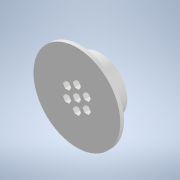
# Autodesk Inventor part: tire vtulka
Saved by Autodesk Inventor 2022 (Build 260153000, 153)
## iProperties
Created: 2023-02-08
Part Number: tire vtulka
Material: Типовые
Document SubType Name: Modeling
Designer: akapu
Density: 1 g/cm^3
Appearance: По умолчанию
Author: akapu
Autodesk Inventor part; units mm, degrees
ref_plane "YZ Plane" through (0, 0, 0) normal (1, 0, 0) x (0, 1, 0)
ref_plane "XZ Plane" through (0, 0, 0) normal (0, 1, 0) x (-1, 0, 0)
ref_plane "XY Plane" through (0, 0, 0) normal (0, 0, 1) x (1, 0, 0)
sketch "Эскиз1" plane through (0, 0, 0) normal (1, 0, 0) x (0, 1, 0)
  line L0 (-3.98, -3) -> (-3.38, 0)
  line L1 (-3.98, -3) -> (-56.02, -3) projected
  line L2 (-4.48, -22.93) -> (-4.48, -3)
  line L3 (-55.52, -22.93) -> (-55.52, -3)
  line L4 (-3.98, -3) -> (-56.02, -3) projected
  line L5 (-56.02, -3) -> (-56.62, 0)
  line L6 (-60, 0) -> (0, 0) projected
  line L7 (-60, 0) -> (-60, -22.93)
  line L8 (0, 0) -> (0, -22.93)
  line L9 (-60, -22.93) -> (0, -22.93) projected
  line L10 (-3.98, -3) -> (-3.98, -3)
  line L11 (-3.98, -3) -> (-3.38, 0)
  line L12 (-56.02, -3) -> (-56.02, -3)
  line L13 (-56.02, -3) -> (-56.62, 0)
  line L14 (-3.38, 0) -> (4.62, 0)
  line L15 (-56.62, 0) -> (-64.62, 0)
  line L16 (-64.62, 0) -> (-64.62, 3)
  line L17 (-64.62, 3) -> (4.62, 3)
  line L18 (4.62, 3) -> (4.62, 0)
  line L19 (-30, -3) -> (-51.25, -3)
  line L20 (-51.25, -3) -> (-8.75, -3)
  line L21 (-8.75, -3) -> (-8.75, -22.93)
  line L22 (-51.25, -3) -> (-51.25, -22.93)
  line L23 (-8.4375, -4) -> (-8.4375, -3)
  line L24 (-8.125, -4) -> (-8.75, -4)
  spline S0 degree 2 poles (-7.5, -3) (-8.8703, -3.1757) (-8.75, -5) knots 0 0 0 1 1 1
  line L25 (-7.5, -3) -> (-8.75, -5)
  line L26 (-7.5, -3) -> (-8.75, -3)
  line L27 (-8.125, -21.93) -> (-8.75, -21.93)
  line L28 (-7.5, -22.93) -> (-8.75, -20.93)
  line L29 (-7.5, -22.93) -> (-8.75, -22.93)
  spline S1 degree 2 poles (-7.5, -22.93) (-8.8703, -22.7543) (-8.75, -20.93) knots 0 0 0 1 1 1
  line L30 (-8.4375, -21.93) -> (-8.4375, -22.93)
  line L31 (-51.875, -4) -> (-51.25, -4)
  line L32 (-52.5, -3) -> (-51.25, -5)
  line L33 (-52.5, -3) -> (-51.25, -3)
  spline S2 degree 2 poles (-52.5, -3) (-51.1297, -3.1757) (-51.25, -5) knots 0 0 0 1 1 1
  line L34 (-51.5625, -4) -> (-51.5625, -3)
  line L35 (-52.5, -22.93) -> (-51.25, -22.93)
  line L36 (-51.5625, -21.93) -> (-51.5625, -22.93)
  line L37 (-51.875, -21.93) -> (-51.25, -21.93)
  line L38 (-52.5, -22.93) -> (-51.25, -20.93)
  spline S3 degree 2 poles (-52.5, -22.93) (-51.1297, -22.7543) (-51.25, -20.93) knots 0 0 0 1 1 1
  line L39 (-8.75, -22.93) -> (-8.75, -15.93)
  line L40 (-8.75, -15.93) -> (-51.25, -15.93)
  line L41 (-30, 3) -> (-30, -22.93)
  line L42 (-8.75, -15.93) -> (-11.75, -15.93)
  line L43 (-30, -15.93) -> (-30, -17.93)
  line L44 (-11.75, -15.93) -> (-13.75, -17.93)
  line L45 (-11.75, -15.93) -> (-8.9216, -15.93) construction
  line L46 (-13.75, -17.93) -> (-30, -17.93)
  point P0 (-8.4375, -3.5)
  point P1 (-8.4375, -22.43)
  point P2 (-51.5625, -3.5)
  point P3 (-51.5625, -22.43)
  point P4 (-30, -15.93)
  dimension "d0" = 0
  dimension "d1" = 0
  dimension "d2" = 8
  dimension "d3" = 8
  dimension "d4" = 3
  dimension "d5" = 21.25
  dimension "d6" = 42.5
  dimension "d11" = 7
  dimension "d13" = 3
  dimension "d14" = 2
  dimension "d15" = 135
  dimension "d20" = 0
  dimension "d21" = 0
  constraints: 86 end point, 14 point on line, 7 perpendicular, 6 midpoint, 4 vertical, 2 horizontal, 1 collinear, 1 equal length, 29 other
  measures "d0" distance of L0.start L10.end
  measures "d1" distance of L1.end L12.end
  measures "d2" distance of L11.end L14.end
  measures "d3" distance of L13.end L15.end
  measures "d4" distance of L15.end L16.end
  measures "d5" distance of L19.start L19.end
  measures "d6" distance of L19.end L20.end
  measures "d11" distance of L29.end L39.end
  measures "d13" distance of L39.end L42.end
  measures "d14" distance of L43.start L43.end
  measures "d15" angle of L44 L45
  measures "d20" distance of L11.end L0.end
  measures "d21" distance of L5.end L13.end
revolve "Вращение1" add sketch "Эскиз1" angle 360 about axis through (0, -30, 3) along (0, 0, -1) contours L41 L1 L5 L6 | L6 L15 L16 L17 L41 | L41 L40 L22 S2 L1 | L22 L31 S2 L34 L1 | L40 L44 L46 L41 | L34 S2 L1 | L22 S2 L31
sketch "Эскиз2" plane through (0, -30, 3) normal (0, 0, 1) x (1, 0, 0)
  circle A0 centre (0, 0) radius 22.5 projected
  line L0 (1.6454, 6.15) -> (3.2909, 9) projected
  line L1 (3.2909, 9) -> (1.6454, 11.85) projected
  line L2 (1.6454, 11.85) -> (-1.6454, 11.85) projected
  line L3 (-1.6454, 11.85) -> (-3.2909, 9) projected
  line L4 (-3.2909, 9) -> (-1.6454, 6.15) projected
  line L5 (-1.6454, 6.15) -> (1.6454, 6.15) projected
  line L6 (-4.5033, 4.5) -> (-6.1488, 7.35) projected
  line L7 (-6.1488, 7.35) -> (-9.4397, 7.35) projected
  line L8 (-9.4397, 7.35) -> (-11.0851, 4.5) projected
  line L9 (-11.0851, 4.5) -> (-9.4397, 1.65) projected
  line L10 (-9.4397, 1.65) -> (-6.1488, 1.65) projected
  line L11 (-6.1488, 1.65) -> (-4.5033, 4.5) projected
  line L12 (-6.1488, -1.65) -> (-9.4397, -1.65) projected
  line L13 (-9.4397, -1.65) -> (-11.0851, -4.5) projected
  line L14 (-11.0851, -4.5) -> (-9.4397, -7.35) projected
  line L15 (-9.4397, -7.35) -> (-6.1488, -7.35) projected
  line L16 (-6.1488, -7.35) -> (-4.5033, -4.5) projected
  line L17 (-4.5033, -4.5) -> (-6.1488, -1.65) projected
  line L18 (-1.6454, -6.15) -> (-3.2909, -9) projected
  line L19 (1.6454, -6.15) -> (-1.6454, -6.15) projected
  line L20 (-3.2909, -9) -> (-1.6454, -11.85) projected
  line L21 (-1.6454, -11.85) -> (1.6454, -11.85) projected
  line L22 (1.6454, -11.85) -> (3.2909, -9) projected
  line L23 (3.2909, -9) -> (1.6454, -6.15) projected
  line L24 (11.0851, -4.5) -> (9.4397, -1.65) projected
  line L25 (9.4397, -1.65) -> (6.1488, -1.65) projected
  line L26 (6.1488, -1.65) -> (4.5033, -4.5) projected
  line L27 (4.5033, -4.5) -> (6.1488, -7.35) projected
  line L28 (6.1488, -7.35) -> (9.4397, -7.35) projected
  line L29 (9.4397, -7.35) -> (11.0851, -4.5) projected
  line L30 (9.4397, 1.65) -> (11.0851, 4.5) projected
  line L31 (6.1488, 1.65) -> (9.4397, 1.65) projected
  line L32 (4.5033, 4.5) -> (6.1488, 1.65) projected
  line L33 (6.1488, 7.35) -> (4.5033, 4.5) projected
  line L34 (9.4397, 7.35) -> (6.1488, 7.35) projected
  line L35 (11.0851, 4.5) -> (9.4397, 7.35) projected
  line L36 (3.2909, 0) -> (1.6454, 2.85) projected
  line L37 (1.6454, 2.85) -> (-1.6454, 2.85) projected
  line L38 (-1.6454, 2.85) -> (-3.2909, 0) projected
  line L39 (-3.2909, 0) -> (-1.6454, -2.85) projected
  line L40 (-1.6454, -2.85) -> (1.6454, -2.85) projected
  line L41 (1.6454, -2.85) -> (3.2909, 0) projected
  circle A1 centre (0, 0) radius 1.7 projected
  circle A2 centre (0, -9) radius 1.7 projected
  circle A3 centre (7.7942, -4.5) radius 1.7 projected
  circle A4 centre (7.7942, 4.5) radius 1.7 projected
  circle A5 centre (0, 9) radius 1.7 projected
  circle A6 centre (-7.7942, 4.5) radius 1.7 projected
  circle A7 centre (-7.7942, -4.5) radius 1.7 projected
  point P0 (0, 30)
extrude "Выдавливание1" cut sketch "Эскиз2" against normal blind 12 contours L5 L4 L3 L2 L1 L0 | L11 L10 L9 L8 L7 L6 | L17 L16 L15 L14 L13 L12 | L19 L23 L22 L21 L20 L18 | L29 L28 L27 L26 L25 L24 | L31 L32 L33 L34 L35 L30 | L41 L40 L39 L38 L37 L36
sketch "Эскиз3" plane through (0, -30, 3) normal (0, 0, 1) x (1, 0, 0)
  circle A0 centre (0, -9) radius 1.7
  circle A1 centre (0, 0) radius 1.7
  circle A2 centre (-7.7942, -4.5) radius 1.7
  circle A3 centre (-7.7942, 4.5) radius 1.7
  circle A4 centre (0, 9) radius 1.7
  circle A5 centre (7.7942, 4.5) radius 1.7
  circle A6 centre (7.7942, -4.5) radius 1.7
  point P0 (0, 30)
extrude "Выдавливание2" cut sketch "Эскиз3" against normal up to surface (25.93 mm away)
